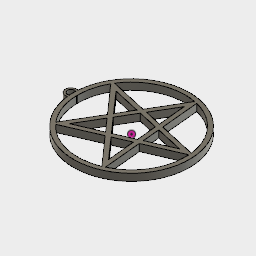
挂件 (Autodesk Fusion 360 design; units mm, degrees)
Autodesk Fusion 360 part; units mm, degrees
sketch "草图1" plane through (0, 0, 0) normal (0, 1, 0) x (1, 0, 0)
sketch "草图2" plane through (0, 0, 0) normal (0, 1, 0) x (1, 0, 0)
  circle A0 centre (0, 0) radius 40.6099
  arc A1 (-32.8609, 18.2939) -> (-28.8479, -24.131) centre (0, 0) ccw
  arc A2 (7.2439, 36.9057) -> (-31.8644, 19.9791) centre (0, 0) ccw
  arc A3 (37.3379, 4.5151) -> (9.1546, 36.4787) centre (0, 0) ccw
  arc A4 (-27.5531, -25.5995) -> (14.0354, -34.8929) centre (0, 0) ccw
  arc A5 (15.8322, -34.1152) -> (37.5223, 2.566) centre (0, 0) ccw
  line L0 (-31.8644, 19.9791) -> (-6.1613, 14.2355)
  line L1 (-26.5994, 15.7286) -> (-7.7668, 11.5202)
  line L2 (-13.3565, -3.8268) -> (-23.1784, -20.4371)
  line L3 (-15.4427, -1.4607) -> (-28.8479, -24.131)
  line L4 (-3.3828, -15.1382) -> (14.0354, -34.8929)
  line L5 (-0.4879, -13.8853) -> (12.2743, -28.3594)
  line L6 (-26.5994, 15.7286) -> (-13.8371, 1.2545)
  line L7 (-11.7509, -1.1115) -> (-2.5741, -11.5193)
  line L8 (-32.8609, 18.2939) -> (-15.4427, -1.4607)
  line L9 (-13.3565, -3.8268) -> (-5.469, -12.7722)
  line L10 (-3.3828, -15.1382) -> (-27.5531, -25.5995)
  line L11 (-5.469, -12.7722) -> (-23.1784, -20.4371)
  line L12 (10.4571, -9.1481) -> (12.2743, -28.3594)
  line L13 (13.352, -7.8952) -> (15.8322, -34.1152)
  line L14 (30.7644, 2.91) -> (13.0549, -4.7548)
  line L15 (10.1601, -6.0078) -> (-2.5741, -11.5193)
  line L16 (37.5223, 2.566) -> (13.352, -7.8952)
  line L17 (10.4571, -9.1481) -> (-0.4879, -13.8853)
  line L18 (-4.6884, 10.8323) -> (8.8534, 7.8063)
  line L19 (11.9318, 7.1184) -> (30.7644, 2.91)
  line L20 (-3.0828, 13.5475) -> (8.5563, 10.9467)
  line L21 (11.6348, 10.2587) -> (37.3379, 4.5151)
  line L22 (6.7391, 30.1579) -> (8.5563, 10.9467)
  line L23 (8.8534, 7.8063) -> (10.1601, -6.0078)
  line L24 (9.1546, 36.4787) -> (11.6348, 10.2587)
  line L25 (11.9318, 7.1184) -> (13.0549, -4.7548)
  line L26 (6.7391, 30.1579) -> (-3.0828, 13.5475)
  line L27 (-4.6884, 10.8323) -> (-11.7509, -1.1115)
  line L28 (7.2439, 36.9057) -> (-6.1613, 14.2355)
  line L29 (-7.7668, 11.5202) -> (-13.8371, 1.2545)
extrude "拉伸1" add sketch "草图2" along normal blind 5 makes body 1
sketch "草图3" plane through (0, 0, 0) normal (0, 1, 0) x (1, 0, 0)
  circle A0 centre (-95, 0) radius 2.5
  circle A1 centre (-95, 0) radius 4
  dimension "d6" = 5
  dimension "d7" = 8
  measures "d6" diameter of A0
  measures "d7" diameter of A1
extrude "拉伸2" add sketch "草图3" along normal blind 5 separate body makes body 2
move_body "移动1" bodies 2 to x (1, 0, 0) y (0, 1, 0) z (0, 0, 1) at (54.5157, 0, 0.7678)
move_body "移动2" bodies 2 to x (1, 0, 0) y (0, 1, 0) z (0, 0, 1) at (-1.1104, 0, 0.0218)
combine "合并1" operation add target body 1 tool bodies 2
